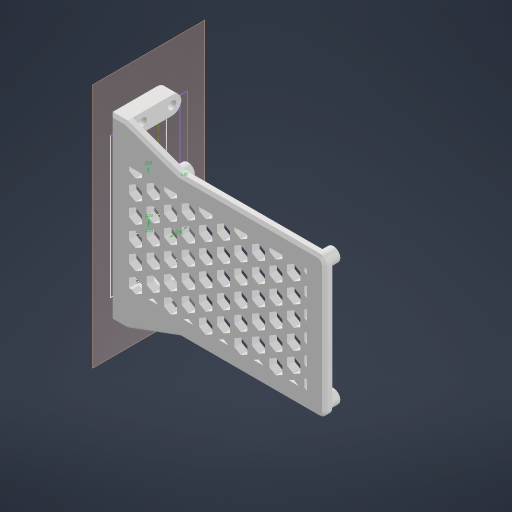
# Autodesk Inventor part: RaspberryPi_baseplate
Saved by Autodesk Inventor 2024 (Build 280153000, 153)
## iProperties
Created: 2025-09-25
Part Number: RaspberryPi_baseplate
Material: Generic
Document SubType Name: Modeling
Designer: kevin
Density: 1 g/cm^3
Appearance: Default
Author: kevin
Autodesk Inventor part; units mm, degrees
(part 1 of 2)
ref_plane "YZ Plane" through (0, 0, 0) normal (1, 0, 0) x (0, 1, 0)
ref_plane "XZ Plane" through (0, 0, 0) normal (0, 1, 0) x (-1, 0, 0)
ref_plane "XY Plane" through (0, 0, 0) normal (0, 0, 1) x (1, 0, 0)
sketch "Sketch1" plane through (0, 0, 0) normal (0, 0, 1) x (1, 0, 0)
  line L0 (-39.5, -28) -> (39.5, -28) projected
  arc A0 (39.5, -28) -> (42.5, -25) centre (39.5, -25) ccw projected
  line L1 (42.5, -25) -> (42.5, 25) projected
  arc A1 (42.5, 25) -> (39.5, 28) centre (39.5, 25) ccw projected
  line L2 (39.5, 28) -> (-39.325, 28) projected
  arc A2 (-39.325, 28) -> (-42.5, 24.825) centre (-39.325, 24.825) ccw projected
  line L3 (-42.5, 24.825) -> (-42.5, -25) projected
  arc A3 (-42.5, -25) -> (-39.5, -28) centre (-39.5, -25) ccw projected
  circle A4 centre (39, 24.5) radius 1.35 construction
  circle A5 centre (39, -24.5) radius 1.35 construction
  circle A6 centre (-19, -24.5) radius 1.35 construction
  circle A7 centre (-19, 24.5) radius 1.35 construction
  circle A8 centre (-19, 24.5) radius 2.75
  circle A9 centre (39, 24.5) radius 2.75
  circle A10 centre (39, -24.5) radius 2.75
  circle A11 centre (-19, -24.5) radius 2.75
  circle A12 centre (-19, -24.5) radius 1.1
  circle A13 centre (-19, 24.5) radius 1.1
  circle A14 centre (39, 24.5) radius 1.1
  circle A15 centre (39, -24.5) radius 1.1
  point P0 (0, 0)
  dimension "d0" = 5.5
  dimension "d1" = 5.5
  dimension "d2" = 5.5
  dimension "d3" = 5.5
  dimension "d4" = 2.2
  dimension "d5" = 2.2
  dimension "d6" = 2.2
  dimension "d7" = 2.2
  constraints: 8 centre point, 8 coincident
  measures "d0" diameter of A8
  measures "d1" diameter of A9
  measures "d2" diameter of A10
  measures "d3" diameter of A11
  measures "d4" diameter of A12
  measures "d5" diameter of A13
  measures "d6" diameter of A14
  measures "d7" diameter of A15
extrude "Extrusion1" add sketch "Sketch1" along normal blind 4 contours A8 | A9 | A10 | A11
sketch "Sketch2" plane through (-19, 24.5, 4) normal (0, 0, 1) x (1, 0, 0)
  circle A0 centre (0, 0) radius 2.75 construction
  circle A1 centre (0, 0) radius 1.1 construction
  circle A2 centre (58, 0) radius 2.75 construction
  circle A3 centre (58, 0) radius 1.1 construction
  circle A4 centre (58, -49) radius 2.75 construction
  circle A5 centre (58, -49) radius 1.1 construction
  circle A6 centre (0, -49) radius 2.75 construction
  circle A7 centre (0, -49) radius 1.1 construction
  line L0 (-20.5, -52.5) -> (58.5, -52.5) projected
  arc A8 (58.5, -52.5) -> (61.5, -49.5) centre (58.5, -49.5) ccw projected
  line L1 (61.5, -49.5) -> (61.5, 0.5) projected
  arc A9 (61.5, 0.5) -> (58.5, 3.5) centre (58.5, 0.5) ccw projected
  line L2 (58.5, 3.5) -> (-20.325, 3.5) projected
  arc A10 (-20.325, 3.5) -> (-23.5, 0.325) centre (-20.325, 0.325) ccw construction
  line L3 (-23.5, 0.325) -> (-23.5, -49.5) projected
  arc A11 (-23.5, -49.5) -> (-20.5, -52.5) centre (-20.5, -49.5) ccw construction
  circle A12 centre (58, 0) radius 1.35 construction
  circle A13 centre (58, -49) radius 1.35 construction
  circle A14 centre (0, -49) radius 1.35 construction
  circle A15 centre (0, 0) radius 1.35 construction
  arc A16 (-3.5, -49) -> (0, -52.5) centre (0, -49) ccw construction
  arc A17 (0, 3.5) -> (-3.5, 0) centre (0, 0) ccw construction
  line L4 (-3.5, 0) -> (-3.5, -49) construction
  line L5 (0, 3.5) -> (58.5, 3.5)
  line L6 (0, -52.5) -> (58.5, -52.5)
  line L7 (54.5, -45.5) -> (3.5, -45.5)
  line L8 (3.5, -45.5) -> (3.5, -3.5) construction
  line L9 (3.5, -3.5) -> (54.5, -3.5)
  line L10 (54.5, -3.5) -> (54.5, -45.5)
  line L11 (3.5, -3.5) -> (54.5, -3.5)
  line L12 (54.5, -45.5) -> (3.5, -45.5)
  line L13 (4.524, -5.8635) -> (7.1369, -4.3549)
  line L14 (7.1369, -4.3549) -> (9.7499, -5.8635)
  line L15 (9.7499, -5.8635) -> (9.7499, -8.8807)
  line L16 (9.7499, -8.8807) -> (7.1369, -10.3893)
  line L17 (7.1369, -10.3893) -> (4.524, -8.8807)
  line L18 (4.524, -8.8807) -> (4.524, -5.8635)
  line L19 (9.7499, -16.8807) -> (7.1369, -18.3893)
  line L20 (9.7499, -13.8635) -> (9.7499, -16.8807)
  line L21 (7.1369, -12.3549) -> (9.7499, -13.8635)
  line L22 (4.524, -13.8635) -> (7.1369, -12.3549)
  line L23 (4.524, -16.8807) -> (4.524, -13.8635)
  line L24 (7.1369, -18.3893) -> (4.524, -16.8807)
  line L25 (9.7499, -24.8807) -> (7.1369, -26.3893)
  line L26 (9.7499, -21.8635) -> (9.7499, -24.8807)
  line L27 (7.1369, -20.3549) -> (9.7499, -21.8635)
  line L28 (4.524, -21.8635) -> (7.1369, -20.3549)
  line L29 (4.524, -24.8807) -> (4.524, -21.8635)
  line L30 (7.1369, -26.3893) -> (4.524, -24.8807)
  line L31 (9.7499, -32.8807) -> (7.1369, -34.3893)
  line L32 (9.7499, -29.8635) -> (9.7499, -32.8807)
  line L33 (7.1369, -28.3549) -> (9.7499, -29.8635)
  line L34 (4.524, -29.8635) -> (7.1369, -28.3549)
  line L35 (4.524, -32.8807) -> (4.524, -29.8635)
  line L36 (7.1369, -34.3893) -> (4.524, -32.8807)
  line L37 (9.7499, -40.8807) -> (7.1369, -42.3893)
  line L38 (9.7499, -37.8635) -> (9.7499, -40.8807)
  line L39 (7.1369, -36.3549) -> (9.7499, -37.8635)
  line L40 (4.524, -37.8635) -> (7.1369, -36.3549)
  line L41 (4.524, -40.8807) -> (4.524, -37.8635)
  line L42 (7.1369, -42.3893) -> (4.524, -40.8807)
  line L43 (16.6781, -12.8807) -> (14.0651, -14.3893)
  line L44 (16.6781, -9.8635) -> (16.6781, -12.8807)
  line L45 (14.0651, -8.3549) -> (16.6781, -9.8635)
  line L46 (11.4522, -9.8635) -> (14.0651, -8.3549)
  line L47 (11.4522, -12.8807) -> (11.4522, -9.8635)
  line L48 (14.0651, -14.3893) -> (11.4522, -12.8807)
  line L49 (16.6781, -20.8807) -> (14.0651, -22.3893)
  line L50 (16.6781, -17.8635) -> (16.6781, -20.8807)
  line L51 (14.0651, -16.3549) -> (16.6781, -17.8635)
  line L52 (11.4522, -17.8635) -> (14.0651, -16.3549)
  line L53 (11.4522, -20.8807) -> (11.4522, -17.8635)
  line L54 (14.0651, -22.3893) -> (11.4522, -20.8807)
  line L55 (16.6781, -28.8807) -> (14.0651, -30.3893)
  line L56 (16.6781, -25.8635) -> (16.6781, -28.8807)
  line L57 (14.0651, -24.3549) -> (16.6781, -25.8635)
  line L58 (11.4522, -25.8635) -> (14.0651, -24.3549)
  line L59 (11.4522, -28.8807) -> (11.4522, -25.8635)
  line L60 (14.0651, -30.3893) -> (11.4522, -28.8807)
  line L61 (16.6781, -36.8807) -> (14.0651, -38.3893)
  line L62 (16.6781, -33.8635) -> (16.6781, -36.8807)
  line L63 (14.0651, -32.3549) -> (16.6781, -33.8635)
  line L64 (11.4522, -33.8635) -> (14.0651, -32.3549)
  line L65 (11.4522, -36.8807) -> (11.4522, -33.8635)
  line L66 (14.0651, -38.3893) -> (11.4522, -36.8807)
  line L67 (16.6781, -44.8807) -> (14.0651, -46.3893)
  line L68 (16.6781, -41.8635) -> (16.6781, -44.8807)
  line L69 (14.0651, -40.3549) -> (16.6781, -41.8635)
  line L70 (11.4522, -41.8635) -> (14.0651, -40.3549)
  line L71 (11.4522, -44.8807) -> (11.4522, -41.8635)
  line L72 (14.0651, -46.3893) -> (11.4522, -44.8807)
  line L73 (16.6781, -4.8807) -> (14.0651, -6.3893)
  line L74 (16.6781, -1.8635) -> (16.6781, -4.8807)
  line L75 (11.4522, -4.8807) -> (11.4522, -1.8635)
  line L76 (14.0651, -0.3549) -> (16.6781, -1.8635) construction
  line L77 (11.4522, -1.8635) -> (14.0651, -0.3549) construction
  line L78 (14.0651, -6.3893) -> (11.4522, -4.8807)
  line L79 (9.7499, -48.8807) -> (7.1369, -50.3893) construction
  line L80 (9.7499, -45.8635) -> (9.7499, -48.8807) construction
  line L81 (7.1369, -44.3549) -> (9.7499, -45.8635)
  line L82 (4.524, -45.8635) -> (7.1369, -44.3549)
  line L83 (4.524, -48.8807) -> (4.524, -45.8635) construction
  line L84 (7.1369, -50.3893) -> (4.524, -48.8807) construction
  line L85 (23.7499, -5.8635) -> (23.7499, -8.8807)
  line L86 (21.1369, -4.3549) -> (23.7499, -5.8635)
  line L87 (18.524, -5.8635) -> (21.1369, -4.3549)
  line L88 (18.524, -8.8807) -> (18.524, -5.8635)
  line L89 (21.1369, -10.3893) -> (18.524, -8.8807)
  line L90 (23.7499, -8.8807) -> (21.1369, -10.3893)
  line L91 (18.524, -40.8807) -> (18.524, -37.8635)
  line L92 (21.1369, -42.3893) -> (18.524, -40.8807)
  line L93 (23.7499, -37.8635) -> (23.7499, -40.8807)
  line L94 (23.7499, -40.8807) -> (21.1369, -42.3893)
  line L95 (25.4522, -20.8807) -> (25.4522, -17.8635)
  line L96 (25.4522, -17.8635) -> (28.0651, -16.3549)
  line L97 (28.0651, -14.3893) -> (25.4522, -12.8807)
  line L98 (30.6781, -12.8807) -> (28.0651, -14.3893)
  line L99 (28.0651, -16.3549) -> (30.6781, -17.8635)
  line L100 (28.0651, -22.3893) -> (25.4522, -20.8807)
  line L101 (30.6781, -17.8635) -> (30.6781, -20.8807)
  line L102 (30.6781, -20.8807) -> (28.0651, -22.3893)
  line L103 (25.4522, -41.8635) -> (28.0651, -40.3549)
  line L104 (28.0651, -40.3549) -> (30.6781, -41.8635)
  line L105 (25.4522, -25.8635) -> (28.0651, -24.3549)
  line L106 (28.0651, -24.3549) -> (30.6781, -25.8635)
  line L107 (30.6781, -25.8635) -> (30.6781, -28.8807)
  line L108 (30.6781, -28.8807) -> (28.0651, -30.3893)
  line L109 (28.0651, -30.3893) -> (25.4522, -28.8807)
  line L110 (28.0651, -32.3549) -> (30.6781, -33.8635)
  line L111 (25.4522, -33.8635) -> (28.0651, -32.3549)
  line L112 (30.6781, -33.8635) -> (30.6781, -36.8807)
  line L113 (25.4522, -36.8807) -> (25.4522, -33.8635)
  line L114 (30.6781, -36.8807) -> (28.0651, -38.3893)
  line L115 (28.0651, -38.3893) -> (25.4522, -36.8807)
  line L116 (25.4522, -28.8807) -> (25.4522, -25.8635)
  line L117 (23.7499, -24.8807) -> (21.1369, -26.3893)
  line L118 (23.7499, -21.8635) -> (23.7499, -24.8807)
  line L119 (21.1369, -20.3549) -> (23.7499, -21.8635)
  line L120 (18.524, -21.8635) -> (21.1369, -20.3549)
  line L121 (18.524, -24.8807) -> (18.524, -21.8635)
  line L122 (21.1369, -26.3893) -> (18.524, -24.8807)
  line L123 (23.7499, -32.8807) -> (21.1369, -34.3893)
  line L124 (18.524, -37.8635) -> (21.1369, -36.3549)
  line L125 (21.1369, -36.3549) -> (23.7499, -37.8635)
  line L126 (21.1369, -34.3893) -> (18.524, -32.8807)
  line L127 (23.7499, -29.8635) -> (23.7499, -32.8807)
  line L128 (18.524, -32.8807) -> (18.524, -29.8635)
  line L129 (21.1369, -28.3549) -> (23.7499, -29.8635)
  line L130 (18.524, -29.8635) -> (21.1369, -28.3549)
  line L131 (23.7499, -16.8807) -> (21.1369, -18.3893)
  line L132 (23.7499, -13.8635) -> (23.7499, -16.8807)
  line L133 (21.1369, -18.3893) -> (18.524, -16.8807)
  line L134 (21.1369, -12.3549) -> (23.7499, -13.8635)
  line L135 (18.524, -16.8807) -> (18.524, -13.8635)
  line L136 (18.524, -13.8635) -> (21.1369, -12.3549)
  line L137 (30.6781, -9.8635) -> (30.6781, -12.8807)
  line L138 (28.0651, -8.3549) -> (30.6781, -9.8635)
  line L139 (25.4522, -9.8635) -> (28.0651, -8.3549)
  line L140 (25.4522, -12.8807) -> (25.4522, -9.8635)
  line L141 (28.0651, -6.3893) -> (25.4522, -4.8807)
  line L142 (30.6781, -4.8807) -> (28.0651, -6.3893)
  line L143 (30.6781, -1.8635) -> (30.6781, -4.8807)
  line L144 (28.0651, -0.3549) -> (30.6781, -1.8635) construction
  line L145 (25.4522, -1.8635) -> (28.0651, -0.3549) construction
  line L146 (25.4522, -4.8807) -> (25.4522, -1.8635)
  line L147 (25.4522, -44.8807) -> (25.4522, -41.8635)
  line L148 (28.0651, -46.3893) -> (25.4522, -44.8807)
  line L149 (30.6781, -44.8807) -> (28.0651, -46.3893)
  line L150 (30.6781, -41.8635) -> (30.6781, -44.8807)
  line L151 (21.1369, -44.3549) -> (23.7499, -45.8635)
  line L152 (18.524, -45.8635) -> (21.1369, -44.3549)
  line L153 (18.524, -48.8807) -> (18.524, -45.8635) construction
  line L154 (21.1369, -50.3893) -> (18.524, -48.8807) construction
  line L155 (23.7499, -48.8807) -> (21.1369, -50.3893) construction
  line L156 (23.7499, -45.8635) -> (23.7499, -48.8807) construction
  line L157 (37.7499, -5.8635) -> (37.7499, -8.8807)
  line L158 (35.1369, -4.3549) -> (37.7499, -5.8635)
  line L159 (32.524, -5.8635) -> (35.1369, -4.3549)
  line L160 (32.524, -8.8807) -> (32.524, -5.8635)
  line L161 (35.1369, -10.3893) -> (32.524, -8.8807)
  line L162 (37.7499, -8.8807) -> (35.1369, -10.3893)
  line L163 (32.524, -40.8807) -> (32.524, -37.8635)
  line L164 (35.1369, -42.3893) -> (32.524, -40.8807)
  line L165 (37.7499, -37.8635) -> (37.7499, -40.8807)
  line L166 (37.7499, -40.8807) -> (35.1369, -42.3893)
  line L167 (39.4522, -20.8807) -> (39.4522, -17.8635)
  line L168 (39.4522, -17.8635) -> (42.0651, -16.3549)
  line L169 (42.0651, -14.3893) -> (39.4522, -12.8807)
  line L170 (44.6781, -12.8807) -> (42.0651, -14.3893)
  line L171 (42.0651, -16.3549) -> (44.6781, -17.8635)
  line L172 (42.0651, -22.3893) -> (39.4522, -20.8807)
  line L173 (44.6781, -17.8635) -> (44.6781, -20.8807)
  line L174 (44.6781, -20.8807) -> (42.0651, -22.3893)
  line L175 (39.4522, -41.8635) -> (42.0651, -40.3549)
  line L176 (42.0651, -40.3549) -> (44.6781, -41.8635)
  line L177 (39.4522, -25.8635) -> (42.0651, -24.3549)
  line L178 (42.0651, -24.3549) -> (44.6781, -25.8635)
  line L179 (44.6781, -25.8635) -> (44.6781, -28.8807)
  line L180 (44.6781, -28.8807) -> (42.0651, -30.3893)
  line L181 (42.0651, -30.3893) -> (39.4522, -28.8807)
  line L182 (42.0651, -32.3549) -> (44.6781, -33.8635)
  line L183 (39.4522, -33.8635) -> (42.0651, -32.3549)
  line L184 (44.6781, -33.8635) -> (44.6781, -36.8807)
  line L185 (39.4522, -36.8807) -> (39.4522, -33.8635)
  line L186 (44.6781, -36.8807) -> (42.0651, -38.3893)
  line L187 (42.0651, -38.3893) -> (39.4522, -36.8807)
  line L188 (39.4522, -28.8807) -> (39.4522, -25.8635)
  line L189 (37.7499, -24.8807) -> (35.1369, -26.3893)
  line L190 (37.7499, -21.8635) -> (37.7499, -24.8807)
  line L191 (35.1369, -20.3549) -> (37.7499, -21.8635)
  line L192 (32.524, -21.8635) -> (35.1369, -20.3549)
  line L193 (32.524, -24.8807) -> (32.524, -21.8635)
  line L194 (35.1369, -26.3893) -> (32.524, -24.8807)
  line L195 (37.7499, -32.8807) -> (35.1369, -34.3893)
  line L196 (32.524, -37.8635) -> (35.1369, -36.3549)
  line L197 (35.1369, -36.3549) -> (37.7499, -37.8635)
  line L198 (35.1369, -34.3893) -> (32.524, -32.8807)
  line L199 (37.7499, -29.8635) -> (37.7499, -32.8807)
  line L200 (32.524, -32.8807) -> (32.524, -29.8635)
  line L201 (35.1369, -28.3549) -> (37.7499, -29.8635)
  line L202 (32.524, -29.8635) -> (35.1369, -28.3549)
  line L203 (37.7499, -16.8807) -> (35.1369, -18.3893)
  line L204 (37.7499, -13.8635) -> (37.7499, -16.8807)
  line L205 (35.1369, -18.3893) -> (32.524, -16.8807)
  line L206 (35.1369, -12.3549) -> (37.7499, -13.8635)
  line L207 (32.524, -16.8807) -> (32.524, -13.8635)
  line L208 (32.524, -13.8635) -> (35.1369, -12.3549)
  line L209 (44.6781, -9.8635) -> (44.6781, -12.8807)
  line L210 (42.0651, -8.3549) -> (44.6781, -9.8635)
  line L211 (39.4522, -9.8635) -> (42.0651, -8.3549)
  line L212 (39.4522, -12.8807) -> (39.4522, -9.8635)
  line L213 (42.0651, -6.3893) -> (39.4522, -4.8807)
  line L214 (44.6781, -4.8807) -> (42.0651, -6.3893)
  line L215 (44.6781, -1.8635) -> (44.6781, -4.8807)
  line L216 (42.0651, -0.3549) -> (44.6781, -1.8635) construction
  line L217 (39.4522, -1.8635) -> (42.0651, -0.3549) construction
  line L218 (39.4522, -4.8807) -> (39.4522, -1.8635)
  line L219 (39.4522, -44.8807) -> (39.4522, -41.8635)
  line L220 (42.0651, -46.3893) -> (39.4522, -44.8807)
  line L221 (44.6781, -44.8807) -> (42.0651, -46.3893)
  line L222 (44.6781, -41.8635) -> (44.6781, -44.8807)
  line L223 (35.1369, -44.3549) -> (37.7499, -45.8635)
  line L224 (32.524, -45.8635) -> (35.1369, -44.3549)
  line L225 (32.524, -48.8807) -> (32.524, -45.8635) construction
  line L226 (35.1369, -50.3893) -> (32.524, -48.8807) construction
  line L227 (37.7499, -48.8807) -> (35.1369, -50.3893) construction
  line L228 (37.7499, -45.8635) -> (37.7499, -48.8807) construction
  line L229 (51.7499, -5.8635) -> (51.7499, -8.8807)
  line L230 (49.1369, -4.3549) -> (51.7499, -5.8635)
  line L231 (46.524, -5.8635) -> (49.1369, -4.3549)
  line L232 (46.524, -8.8807) -> (46.524, -5.8635)
  line L233 (49.1369, -10.3893) -> (46.524, -8.8807)
  line L234 (51.7499, -8.8807) -> (49.1369, -10.3893)
  line L235 (46.524, -40.8807) -> (46.524, -37.8635)
  line L236 (49.1369, -42.3893) -> (46.524, -40.8807)
  line L237 (51.7499, -37.8635) -> (51.7499, -40.8807)
  line L238 (51.7499, -40.8807) -> (49.1369, -42.3893)
  line L239 (53.4522, -20.8807) -> (53.4522, -17.8635)
  line L240 (53.4522, -17.8635) -> (56.0651, -16.3549)
  line L241 (56.0651, -14.3893) -> (53.4522, -12.8807)
  line L242 (58.6781, -12.8807) -> (56.0651, -14.3893) construction
  line L243 (56.0651, -16.3549) -> (58.6781, -17.8635) construction
  line L244 (56.0651, -22.3893) -> (53.4522, -20.8807)
  line L245 (58.6781, -17.8635) -> (58.6781, -20.8807) construction
  line L246 (58.6781, -20.8807) -> (56.0651, -22.3893) construction
  line L247 (53.4522, -41.8635) -> (56.0651, -40.3549)
  line L248 (56.0651, -40.3549) -> (58.6781, -41.8635) construction
  line L249 (53.4522, -25.8635) -> (56.0651, -24.3549)
  line L250 (56.0651, -24.3549) -> (58.6781, -25.8635) construction
  line L251 (58.6781, -25.8635) -> (58.6781, -28.8807) construction
  line L252 (58.6781, -28.8807) -> (56.0651, -30.3893) construction
  line L253 (56.0651, -30.3893) -> (53.4522, -28.8807)
  line L254 (56.0651, -32.3549) -> (58.6781, -33.8635) construction
  line L255 (53.4522, -33.8635) -> (56.0651, -32.3549)
  line L256 (58.6781, -33.8635) -> (58.6781, -36.8807) construction
  line L257 (53.4522, -36.8807) -> (53.4522, -33.8635)
  line L258 (58.6781, -36.8807) -> (56.0651, -38.3893) construction
  line L259 (56.0651, -38.3893) -> (53.4522, -36.8807)
  line L260 (53.4522, -28.8807) -> (53.4522, -25.8635)
  line L261 (51.7499, -24.8807) -> (49.1369, -26.3893)
  line L262 (51.7499, -21.8635) -> (51.7499, -24.8807)
  line L263 (49.1369, -20.3549) -> (51.7499, -21.8635)
  line L264 (46.524, -21.8635) -> (49.1369, -20.3549)
  line L265 (46.524, -24.8807) -> (46.524, -21.8635)
  line L266 (49.1369, -26.3893) -> (46.524, -24.8807)
  line L267 (51.7499, -32.8807) -> (49.1369, -34.3893)
  line L268 (46.524, -37.8635) -> (49.1369, -36.3549)
  line L269 (49.1369, -36.3549) -> (51.7499, -37.8635)
  line L270 (49.1369, -34.3893) -> (46.524, -32.8807)
  line L271 (51.7499, -29.8635) -> (51.7499, -32.8807)
  line L272 (46.524, -32.8807) -> (46.524, -29.8635)
  line L273 (49.1369, -28.3549) -> (51.7499, -29.8635)
  line L274 (46.524, -29.8635) -> (49.1369, -28.3549)
  line L275 (51.7499, -16.8807) -> (49.1369, -18.3893)
  line L276 (51.7499, -13.8635) -> (51.7499, -16.8807)
  line L277 (49.1369, -18.3893) -> (46.524, -16.8807)
  line L278 (49.1369, -12.3549) -> (51.7499, -13.8635)
  line L279 (46.524, -16.8807) -> (46.524, -13.8635)
  line L280 (46.524, -13.8635) -> (49.1369, -12.3549)
  line L281 (58.6781, -9.8635) -> (58.6781, -12.8807) construction
  line L282 (56.0651, -8.3549) -> (58.6781, -9.8635) construction
  line L283 (53.4522, -9.8635) -> (56.0651, -8.3549)
  line L284 (53.4522, -12.8807) -> (53.4522, -9.8635)
  line L285 (56.0651, -6.3893) -> (53.4522, -4.8807)
  line L286 (58.6781, -4.8807) -> (56.0651, -6.3893) construction
  line L287 (58.6781, -1.8635) -> (58.6781, -4.8807) construction
  line L288 (56.0651, -0.3549) -> (58.6781, -1.8635)
  line L289 (53.4522, -1.8635) -> (56.0651, -0.3549)
  line L290 (53.4522, -4.8807) -> (53.4522, -1.8635)
  line L291 (53.4522, -44.8807) -> (53.4522, -41.8635)
  line L292 (56.0651, -46.3893) -> (53.4522, -44.8807)
  line L293 (58.6781, -44.8807) -> (56.0651, -46.3893)
  line L294 (58.6781, -41.8635) -> (58.6781, -44.8807) construction
  line L295 (49.1369, -44.3549) -> (51.7499, -45.8635)
  line L296 (46.524, -45.8635) -> (49.1369, -44.3549)
  line L297 (46.524, -48.8807) -> (46.524, -45.8635) construction
  line L298 (49.1369, -50.3893) -> (46.524, -48.8807) construction
  line L299 (51.7499, -48.8807) -> (49.1369, -50.3893) construction
  line L300 (51.7499, -45.8635) -> (51.7499, -48.8807) construction
  line L301 (65.7499, -5.8635) -> (65.7499, -8.8807) construction
  line L302 (63.1369, -4.3549) -> (65.7499, -5.8635) construction
  line L303 (60.524, -5.8635) -> (63.1369, -4.3549) construction
  line L304 (60.524, -8.8807) -> (60.524, -5.8635)
  line L305 (63.1369, -10.3893) -> (60.524, -8.8807) construction
  line L306 (65.7499, -8.8807) -> (63.1369, -10.3893) construction
  line L307 (60.524, -40.8807) -> (60.524, -37.8635)
  line L308 (63.1369, -42.3893) -> (60.524, -40.8807) construction
  line L309 (65.7499, -37.8635) -> (65.7499, -40.8807) construction
  line L310 (65.7499, -40.8807) -> (63.1369, -42.3893) construction
  line L311 (67.4522, -20.8807) -> (67.4522, -17.8635) construction
  line L312 (67.4522, -17.8635) -> (70.0651, -16.3549) construction
  line L313 (70.0651, -14.3893) -> (67.4522, -12.8807) construction
  line L314 (72.6781, -12.8807) -> (70.0651, -14.3893) construction
  line L315 (70.0651, -16.3549) -> (72.6781, -17.8635) construction
  line L316 (70.0651, -22.3893) -> (67.4522, -20.8807) construction
  line L317 (72.6781, -17.8635) -> (72.6781, -20.8807) construction
  line L318 (72.6781, -20.8807) -> (70.0651, -22.3893) construction
  line L319 (67.4522, -41.8635) -> (70.0651, -40.3549) construction
  line L320 (70.0651, -40.3549) -> (72.6781, -41.8635) construction
  line L321 (67.4522, -25.8635) -> (70.0651, -24.3549) construction
  line L322 (70.0651, -24.3549) -> (72.6781, -25.8635) construction
  line L323 (72.6781, -25.8635) -> (72.6781, -28.8807) construction
  line L324 (72.6781, -28.8807) -> (70.0651, -30.3893) construction
  line L325 (70.0651, -30.3893) -> (67.4522, -28.8807) construction
  line L326 (70.0651, -32.3549) -> (72.6781, -33.8635) construction
  line L327 (67.4522, -33.8635) -> (70.0651, -32.3549) construction
  line L328 (72.6781, -33.8635) -> (72.6781, -36.8807) construction
  line L329 (67.4522, -36.8807) -> (67.4522, -33.8635) construction
  line L330 (72.6781, -36.8807) -> (70.0651, -38.3893) construction
  line L331 (70.0651, -38.3893) -> (67.4522, -36.8807) construction
  line L332 (67.4522, -28.8807) -> (67.4522, -25.8635) construction
  line L333 (65.7499, -24.8807) -> (63.1369, -26.3893) construction
  line L334 (65.7499, -21.8635) -> (65.7499, -24.8807) construction
  line L335 (63.1369, -20.3549) -> (65.7499, -21.8635) construction
  line L336 (60.524, -21.8635) -> (63.1369, -20.3549) construction
  line L337 (60.524, -24.8807) -> (60.524, -21.8635)
  line L338 (63.1369, -26.3893) -> (60.524, -24.8807) construction
  line L339 (65.7499, -32.8807) -> (63.1369, -34.3893) construction
  line L340 (60.524, -37.8635) -> (63.1369, -36.3549) construction
  line L341 (63.1369, -36.3549) -> (65.7499, -37.8635) construction
  line L342 (63.1369, -34.3893) -> (60.524, -32.8807) construction
  line L343 (65.7499, -29.8635) -> (65.7499, -32.8807) construction
  line L344 (60.524, -32.8807) -> (60.524, -29.8635)
  line L345 (63.1369, -28.3549) -> (65.7499, -29.8635) construction
  line L346 (60.524, -29.8635) -> (63.1369, -28.3549) construction
  line L347 (65.7499, -16.8807) -> (63.1369, -18.3893) construction
  line L348 (65.7499, -13.8635) -> (65.7499, -16.8807) construction
  line L349 (63.1369, -18.3893) -> (60.524, -16.8807) construction
  line L350 (63.1369, -12.3549) -> (65.7499, -13.8635) construction
  line L351 (60.524, -16.8807) -> (60.524, -13.8635)
  line L352 (60.524, -13.8635) -> (63.1369, -12.3549) construction
  line L353 (72.6781, -9.8635) -> (72.6781, -12.8807) construction
  line L354 (70.0651, -8.3549) -> (72.6781, -9.8635) construction
  line L355 (67.4522, -9.8635) -> (70.0651, -8.3549) construction
  line L356 (67.4522, -12.8807) -> (67.4522, -9.8635) construction
  line L357 (70.0651, -6.3893) -> (67.4522, -4.8807) construction
  line L358 (72.6781, -4.8807) -> (70.0651, -6.3893) construction
  line L359 (72.6781, -1.8635) -> (72.6781, -4.8807) construction
  line L360 (70.0651, -0.3549) -> (72.6781, -1.8635) construction
  line L361 (67.4522, -1.8635) -> (70.0651, -0.3549) construction
  line L362 (67.4522, -4.8807) -> (67.4522, -1.8635) construction
  line L363 (67.4522, -44.8807) -> (67.4522, -41.8635) construction
  line L364 (70.0651, -46.3893) -> (67.4522, -44.8807) construction
  line L365 (72.6781, -44.8807) -> (70.0651, -46.3893) construction
  line L366 (72.6781, -41.8635) -> (72.6781, -44.8807) construction
  line L367 (63.1369, -44.3549) -> (65.7499, -45.8635) construction
  line L368 (60.524, -45.8635) -> (63.1369, -44.3549) construction
  line L369 (60.524, -48.8807) -> (60.524, -45.8635)
  line L370 (63.1369, -50.3893) -> (60.524, -48.8807) construction
  line L371 (65.7499, -48.8807) -> (63.1369, -50.3893) construction
  line L372 (65.7499, -45.8635) -> (65.7499, -48.8807) construction
  line L373 (79.7499, -5.8635) -> (79.7499, -8.8807) construction
  line L374 (77.1369, -4.3549) -> (79.7499, -5.8635) construction
  line L375 (74.524, -5.8635) -> (77.1369, -4.3549) construction
  line L376 (74.524, -8.8807) -> (74.524, -5.8635) construction
  line L377 (77.1369, -10.3893) -> (74.524, -8.8807) construction
  line L378 (79.7499, -8.8807) -> (77.1369, -10.3893) construction
  line L379 (74.524, -40.8807) -> (74.524, -37.8635) construction
  line L380 (77.1369, -42.3893) -> (74.524, -40.8807) construction
  line L381 (79.7499, -37.8635) -> (79.7499, -40.8807) construction
  line L382 (79.7499, -40.8807) -> (77.1369, -42.3893) construction
  line L383 (81.4522, -20.8807) -> (81.4522, -17.8635) construction
  line L384 (81.4522, -17.8635) -> (84.0651, -16.3549) construction
  line L385 (84.0651, -14.3893) -> (81.4522, -12.8807) construction
  line L386 (86.6781, -12.8807) -> (84.0651, -14.3893) construction
  line L387 (84.0651, -16.3549) -> (86.6781, -17.8635) construction
  line L388 (84.0651, -22.3893) -> (81.4522, -20.8807) construction
  line L389 (86.6781, -17.8635) -> (86.6781, -20.8807) construction
  line L390 (86.6781, -20.8807) -> (84.0651, -22.3893) construction
  line L391 (81.4522, -41.8635) -> (84.0651, -40.3549) construction
  line L392 (84.0651, -40.3549) -> (86.6781, -41.8635) construction
  line L393 (81.4522, -25.8635) -> (84.0651, -24.3549) construction
  line L394 (84.0651, -24.3549) -> (86.6781, -25.8635) construction
  line L395 (86.6781, -25.8635) -> (86.6781, -28.8807) construction
  line L396 (86.6781, -28.8807) -> (84.0651, -30.3893) construction
  line L397 (84.0651, -30.3893) -> (81.4522, -28.8807) construction
  line L398 (84.0651, -32.3549) -> (86.6781, -33.8635) construction
  line L399 (81.4522, -33.8635) -> (84.0651, -32.3549) construction
  line L400 (86.6781, -33.8635) -> (86.6781, -36.8807) construction
  line L401 (81.4522, -36.8807) -> (81.4522, -33.8635) construction
  line L402 (86.6781, -36.8807) -> (84.0651, -38.3893) construction
  line L403 (84.0651, -38.3893) -> (81.4522, -36.8807) construction
  line L404 (81.4522, -28.8807) -> (81.4522, -25.8635) construction
  line L405 (79.7499, -24.8807) -> (77.1369, -26.3893) construction
  line L406 (79.7499, -21.8635) -> (79.7499, -24.8807) construction
  line L407 (77.1369, -20.3549) -> (79.7499, -21.8635) construction
  line L408 (74.524, -21.8635) -> (77.1369, -20.3549) construction
  line L409 (74.524, -24.8807) -> (74.524, -21.8635) construction
  line L410 (77.1369, -26.3893) -> (74.524, -24.8807) construction
  line L411 (79.7499, -32.8807) -> (77.1369, -34.3893) construction
  line L412 (74.524, -37.8635) -> (77.1369, -36.3549) construction
  line L413 (77.1369, -36.3549) -> (79.7499, -37.8635) construction
  line L414 (77.1369, -34.3893) -> (74.524, -32.8807) construction
  line L415 (79.7499, -29.8635) -> (79.7499, -32.8807) construction
  line L416 (74.524, -32.8807) -> (74.524, -29.8635) construction
  line L417 (77.1369, -28.3549) -> (79.7499, -29.8635) construction
  line L418 (74.524, -29.8635) -> (77.1369, -28.3549) construction
  line L419 (79.7499, -16.8807) -> (77.1369, -18.3893) construction
  line L420 (79.7499, -13.8635) -> (79.7499, -16.8807) construction
  line L421 (77.1369, -18.3893) -> (74.524, -16.8807) construction
  line L422 (77.1369, -12.3549) -> (79.7499, -13.8635) construction
  line L423 (74.524, -16.8807) -> (74.524, -13.8635) construction
  line L424 (74.524, -13.8635) -> (77.1369, -12.3549) construction
  line L425 (86.6781, -9.8635) -> (86.6781, -12.8807) construction
  line L426 (84.0651, -8.3549) -> (86.6781, -9.8635) construction
  line L427 (81.4522, -9.8635) -> (84.0651, -8.3549) construction
  line L428 (81.4522, -12.8807) -> (81.4522, -9.8635) construction
  line L429 (84.0651, -6.3893) -> (81.4522, -4.8807) construction
  line L430 (86.6781, -4.8807) -> (84.0651, -6.3893) construction
  line L431 (86.6781, -1.8635) -> (86.6781, -4.8807) construction
  line L432 (84.0651, -0.3549) -> (86.6781, -1.8635) construction
  line L433 (81.4522, -1.8635) -> (84.0651, -0.3549) construction
  line L434 (81.4522, -4.8807) -> (81.4522, -1.8635) construction
  line L435 (81.4522, -44.8807) -> (81.4522, -41.8635) construction
  line L436 (84.0651, -46.3893) -> (81.4522, -44.8807) construction
  line L437 (86.6781, -44.8807) -> (84.0651, -46.3893) construction
  line L438 (86.6781, -41.8635) -> (86.6781, -44.8807) construction
  line L439 (77.1369, -44.3549) -> (79.7499, -45.8635) construction
  line L440 (74.524, -45.8635) -> (77.1369, -44.3549) construction
  line L441 (74.524, -48.8807) -> (74.524, -45.8635) construction
  line L442 (77.1369, -50.3893) -> (74.524, -48.8807) construction
  line L443 (79.7499, -48.8807) -> (77.1369, -50.3893) construction
  line L444 (79.7499, -45.8635) -> (79.7499, -48.8807) construction
  line L445 (-13.5, 3.5) -> (-13.5, -52.5) construction
  line L446 (-13.5, 3.5) -> (0, 3.5)
  line L447 (-23.5, -52.5) -> (0, -52.5)
  line L448 (-16.5, -45.5) -> (-16.5, -3.5)
  line L449 (-16.5, -3.5) -> (54.5, -3.5)
  line L450 (54.5, -3.5) -> (54.5, -45.5)
  line L451 (54.5, -45.5) -> (-16.5, -45.5)
  line L452 (-23.5, -15.3721) -> (-23.5, 3.5)
  line L453 (-16.7764, 3.5) -> (-23.5, 3.5)
  line L454 (-23.5, -49.5) -> (-23.5, -52.5)
  line L455 (2.6781, -9.8635) -> (2.6781, -12.8807)
  line L456 (2.6781, -12.8807) -> (0.0651, -14.3893)
  line L457 (0.0651, -8.3549) -> (2.6781, -9.8635)
  line L458 (0.0651, -16.3549) -> (2.6781, -17.8635)
  line L459 (2.6781, -17.8635) -> (2.6781, -20.8807)
  line L460 (2.6781, -20.8807) -> (0.0651, -22.3893)
  line L461 (-2.5478, -9.8635) -> (0.0651, -8.3549)
  line L462 (-2.5478, -12.8807) -> (-2.5478, -9.8635)
  line L463 (0.0651, -14.3893) -> (-2.5478, -12.8807)
  line L464 (0.0651, -22.3893) -> (-2.5478, -20.8807)
  line L465 (-2.5478, -20.8807) -> (-2.5478, -17.8635)
  line L466 (-2.5478, -17.8635) -> (0.0651, -16.3549)
  line L467 (-4.2501, -24.8807) -> (-6.8631, -26.3893)
  line L468 (-4.2501, -13.8635) -> (-4.2501, -16.8807)
  line L469 (-6.8631, -12.3549) -> (-4.2501, -13.8635)
  line L470 (-4.2501, -16.8807) -> (-6.8631, -18.3893)
  line L471 (-9.476, -8.8807) -> (-9.476, -5.8635)
  line L472 (-6.8631, -10.3893) -> (-9.476, -8.8807)
  line L473 (-6.8631, -18.3893) -> (-9.476, -16.8807)
  line L474 (-9.476, -16.8807) -> (-9.476, -13.8635)
  line L475 (-9.476, -13.8635) -> (-6.8631, -12.3549)
  line L476 (-4.2501, -5.8635) -> (-4.2501, -8.8807)
  line L477 (-6.8631, -4.3549) -> (-4.2501, -5.8635)
  line L478 (-4.2501, -8.8807) -> (-6.8631, -10.3893)
  line L479 (-9.476, -5.8635) -> (-6.8631, -4.3549)
  line L480 (2.6781, -25.8635) -> (2.6781, -28.8807)
  line L481 (0.0651, -24.3549) -> (2.6781, -25.8635)
  line L482 (2.6781, -28.8807) -> (0.0651, -30.3893)
  line L483 (-2.5478, -25.8635) -> (0.0651, -24.3549)
  line L484 (2.6781, -33.8635) -> (2.6781, -36.8807)
  line L485 (0.0651, -32.3549) -> (2.6781, -33.8635)
  line L486 (-2.5478, -28.8807) -> (-2.5478, -25.8635)
  line L487 (0.0651, -30.3893) -> (-2.5478, -28.8807)
  line L488 (-2.5478, -33.8635) -> (0.0651, -32.3549)
  line L489 (-2.5478, -36.8807) -> (-2.5478, -33.8635)
  line L490 (-6.8631, -26.3893) -> (-9.476, -24.8807)
  line L491 (-4.2501, -21.8635) -> (-4.2501, -24.8807)
  line L492 (-4.2501, -29.8635) -> (-4.2501, -32.8807)
  line L493 (-4.2501, -32.8807) -> (-6.8631, -34.3893)
  line L494 (-6.8631, -20.3549) -> (-4.2501, -21.8635)
  line L495 (-6.8631, -28.3549) -> (-4.2501, -29.8635)
  line L496 (-9.476, -29.8635) -> (-6.8631, -28.3549)
  line L497 (-9.476, -24.8807) -> (-9.476, -21.8635)
  line L498 (-9.476, -21.8635) -> (-6.8631, -20.3549)
  line L499 (-4.2501, -37.8635) -> (-4.2501, -40.8807)
  line L500 (-6.8631, -36.3549) -> (-4.2501, -37.8635)
  line L501 (-4.2501, -40.8807) -> (-6.8631, -42.3893)
  line L502 (-9.476, -32.8807) -> (-9.476, -29.8635)
  line L503 (-6.8631, -34.3893) -> (-9.476, -32.8807)
  line L504 (-9.476, -37.8635) -> (-6.8631, -36.3549)
  line L505 (-9.476, -40.8807) -> (-9.476, -37.8635)
  line L506 (-6.8631, -42.3893) -> (-9.476, -40.8807)
  line L507 (2.6781, -36.8807) -> (0.0651, -38.3893)
  line L508 (0.0651, -38.3893) -> (-2.5478, -36.8807)
  line L509 (2.6781, -44.8807) -> (0.0651, -46.3893)
  line L510 (2.6781, -41.8635) -> (2.6781, -44.8807)
  line L511 (0.0651, -40.3549) -> (2.6781, -41.8635)
  line L512 (-2.5478, -41.8635) -> (0.0651, -40.3549)
  line L513 (-2.5478, -44.8807) -> (-2.5478, -41.8635)
  line L514 (0.0651, -46.3893) -> (-2.5478, -44.8807)
  line L515 (-6.8631, -44.3549) -> (-4.2501, -45.8635)
  line L516 (2.6781, -4.8807) -> (0.0651, -6.3893)
  line L517 (0.0651, -6.3893) -> (-2.5478, -4.8807)
  line L518 (2.6781, -1.8635) -> (2.6781, -4.8807)
  line L519 (-2.5478, -4.8807) -> (-2.5478, -1.8635)
  line L520 (0.0651, -0.3549) -> (2.6781, -1.8635) construction
  line L521 (-2.5478, -1.8635) -> (0.0651, -0.3549) construction
  line L522 (4.524, -16.8807) -> (4.524, -13.8635)
  line L523 (4.524, -8.8807) -> (4.524, -5.8635)
  line L524 (-9.476, -45.8635) -> (-6.8631, -44.3549)
  line L525 (-9.476, -48.8807) -> (-9.476, -45.8635) construction
  line L526 (-4.2501, -45.8635) -> (-4.2501, -48.8807) construction
  line L527 (-4.2501, -48.8807) -> (-6.8631, -50.3893) construction
  line L528 (-6.8631, -50.3893) -> (-9.476, -48.8807) construction
  line L529 (-11.3219, -9.8635) -> (-11.3219, -12.8807)
  line L530 (-11.3219, -12.8807) -> (-13.9349, -14.3893)
  line L531 (-13.9349, -8.3549) -> (-11.3219, -9.8635)
  line L532 (-13.9349, -16.3549) -> (-11.3219, -17.8635)
  line L533 (-11.3219, -17.8635) -> (-11.3219, -20.8807)
  line L534 (-11.3219, -20.8807) -> (-13.9349, -22.3893)
  line L535 (-16.5478, -9.8635) -> (-13.9349, -8.3549)
  line L536 (-16.5478, -12.8807) -> (-16.5478, -9.8635)
  line L537 (-13.9349, -14.3893) -> (-16.5478, -12.8807)
  line L538 (-13.9349, -22.3893) -> (-16.5478, -20.8807)
  line L539 (-16.5478, -20.8807) -> (-16.5478, -17.8635)
  line L540 (-16.5478, -17.8635) -> (-13.9349, -16.3549)
  line L541 (-18.2501, -24.8807) -> (-20.8631, -26.3893) construction
  line L542 (-18.2501, -13.8635) -> (-18.2501, -16.8807) construction
  line L543 (-20.8631, -12.3549) -> (-18.2501, -13.8635) construction
  line L544 (-18.2501, -16.8807) -> (-20.8631, -18.3893) construction
  line L545 (-23.476, -8.8807) -> (-23.476, -5.8635)
  line L546 (-20.8631, -10.3893) -> (-23.476, -8.8807) construction
  line L547 (-20.8631, -18.3893) -> (-23.476, -16.8807) construction
  line L548 (-23.476, -16.8807) -> (-23.476, -13.8635)
  line L549 (-23.476, -13.8635) -> (-20.8631, -12.3549) construction
  line L550 (-18.2501, -5.8635) -> (-18.2501, -8.8807) construction
  line L551 (-20.8631, -4.3549) -> (-18.2501, -5.8635) construction
  line L552 (-18.2501, -8.8807) -> (-20.8631, -10.3893) construction
  line L553 (-23.476, -5.8635) -> (-20.8631, -4.3549) construction
  line L554 (-11.3219, -25.8635) -> (-11.3219, -28.8807)
  line L555 (-13.9349, -24.3549) -> (-11.3219, -25.8635)
  line L556 (-11.3219, -28.8807) -> (-13.9349, -30.3893)
  line L557 (-16.5478, -25.8635) -> (-13.9349, -24.3549)
  line L558 (-11.3219, -33.8635) -> (-11.3219, -36.8807)
  line L559 (-13.9349, -32.3549) -> (-11.3219, -33.8635)
  line L560 (-16.5478, -28.8807) -> (-16.5478, -25.8635)
  line L561 (-13.9349, -30.3893) -> (-16.5478, -28.8807)
  line L562 (-16.5478, -33.8635) -> (-13.9349, -32.3549)
  line L563 (-16.5478, -36.8807) -> (-16.5478, -33.8635)
  line L564 (-20.8631, -26.3893) -> (-23.476, -24.8807) construction
  line L565 (-18.2501, -21.8635) -> (-18.2501, -24.8807)
  line L566 (-18.2501, -29.8635) -> (-18.2501, -32.8807) construction
  line L567 (-18.2501, -32.8807) -> (-20.8631, -34.3893) construction
  line L568 (-20.8631, -20.3549) -> (-18.2501, -21.8635) construction
  line L569 (-20.8631, -28.3549) -> (-18.2501, -29.8635) construction
  line L570 (-23.476, -29.8635) -> (-20.8631, -28.3549) construction
  line L571 (-23.476, -24.8807) -> (-23.476, -21.8635)
  line L572 (-23.476, -21.8635) -> (-20.8631, -20.3549) construction
  line L573 (-18.2501, -37.8635) -> (-18.2501, -40.8807) construction
  line L574 (-20.8631, -36.3549) -> (-18.2501, -37.8635) construction
  line L575 (-18.2501, -40.8807) -> (-20.8631, -42.3893) construction
  line L576 (-23.476, -32.8807) -> (-23.476, -29.8635)
  line L577 (-20.8631, -34.3893) -> (-23.476, -32.8807) construction
  line L578 (-23.476, -37.8635) -> (-20.8631, -36.3549) construction
  line L579 (-23.476, -40.8807) -> (-23.476, -37.8635)
  line L580 (-20.8631, -42.3893) -> (-23.476, -40.8807) construction
  line L581 (-11.3219, -36.8807) -> (-13.9349, -38.3893)
  line L582 (-13.9349, -38.3893) -> (-16.5478, -36.8807)
  line L583 (-11.3219, -44.8807) -> (-13.9349, -46.3893)
  line L584 (-11.3219, -41.8635) -> (-11.3219, -44.8807)
  line L585 (-13.9349, -40.3549) -> (-11.3219, -41.8635)
  line L586 (-16.5478, -41.8635) -> (-13.9349, -40.3549)
  line L587 (-16.5478, -44.8807) -> (-16.5478, -41.8635)
  line L588 (-13.9349, -46.3893) -> (-16.5478, -44.8807)
  line L589 (-20.8631, -44.3549) -> (-18.2501, -45.8635) construction
  line L590 (-11.3219, -4.8807) -> (-13.9349, -6.3893)
  line L591 (-13.9349, -6.3893) -> (-16.5478, -4.8807)
  line L592 (-11.3219, -1.8635) -> (-11.3219, -4.8807)
  line L593 (-16.5478, -4.8807) -> (-16.5478, -1.8635)
  line L594 (-13.9349, -0.3549) -> (-11.3219, -1.8635) construction
  line L595 (-16.5478, -1.8635) -> (-13.9349, -0.3549) construction
  line L596 (-9.476, -16.8807) -> (-9.476, -13.8635)
  line L597 (-9.476, -8.8807) -> (-9.476, -5.8635)
  line L598 (-23.476, -45.8635) -> (-20.8631, -44.3549) construction
  line L599 (-23.476, -48.8807) -> (-23.476, -45.8635)
  line L600 (-18.2501, -45.8635) -> (-18.2501, -48.8807) construction
  line L601 (-18.2501, -48.8807) -> (-20.8631, -50.3893) construction
  line L602 (-20.8631, -50.3893) -> (-23.476, -48.8807) construction
  line L603 (-23.5, -52.5) -> (-24, -52.5)
  line L604 (-24, -52.5) -> (-24, 3.5)
  line L605 (-24, 3.5) -> (-23.5, 3.5)
  point P0 (0, 3.5)
  point P1 (0, -52.5)
  point P2 (7.1369, -7.3721)
  point P3 (5.1535, -45.5)
  point P4 (9.1204, -45.5)
  point P5 (19.1535, -45.5)
  point P6 (23.1204, -45.5)
  point P7 (26.5249, -45.5)
  point P8 (29.6054, -45.5)
  point P9 (33.1535, -45.5)
  point P10 (37.1204, -45.5)
  point P11 (47.1535, -45.5)
  point P12 (51.1204, -45.5)
  point P13 (54.5, -45.4856)
  point P14 (54.5, -41.2585)
  point P15 (54.5, -37.4856)
  point P16 (54.5, -33.2585)
  point P17 (54.5, -29.4856)
  point P18 (54.5, -25.2585)
  point P19 (54.5, -21.4856)
  point P20 (54.5, -17.2585)
  point P21 (54.5, -13.4856)
  point P22 (54.5, -9.2585)
  point P23 (54.5, -5.4856)
  point P24 (53.4522, -3.5)
  point P25 (44.6781, -3.5)
  point P26 (39.4522, -3.5)
  point P27 (30.6781, -3.5)
  point P28 (25.4522, -3.5)
  point P29 (16.6781, -3.5)
  point P30 (11.4522, -3.5)
  point P31 (-10.5, -45.5)
  point P32 (-6.8631, -7.3721)
  point P33 (-24.5, -45.5)
  point P34 (-20.8631, -7.3721)
  point P35 (12.5249, -45.5)
  point P36 (15.6054, -45.5)
  point P37 (-23.5, 0.325)
  point P38 (40.5249, -45.5)
  point P39 (43.6054, -45.5)
  point P40 (-2.5478, -3.5)
  point P41 (2.6781, -3.5)
  point P42 (-16.5, -4.9083)
  point P43 (-11.3219, -3.5)
  point P44 (-16.5, -12.9083)
  point P45 (-16.5, -9.8359)
  point P46 (-12.3946, -45.5)
  point P47 (-15.4751, -45.5)
  point P48 (-4.8796, -45.5)
  point P49 (-8.8465, -45.5)
  point P50 (-1.4751, -45.5)
  point P51 (1.6054, -45.5)
  point P52 (-16.5, -44.9083)
  dimension "d16" = 7
  dimension "d17" = 7
  dimension "d18" = 51
  dimension "d21" = 8
  dimension "d24" = 8
  dimension "d29" = 8
  dimension "d36" = 8
  dimension "d43" = 14
  dimension "d48" = 10
  dimension "d50" = 7
  dimension "d53" = 14
  dimension "d60" = 0.5
  constraints: 1204 end point, 7 point on line, 6 collinear, 6 vertical, 5 horizontal, 4 point on circle, 3 perpendicular, 2 centre point, 2 tangent, 1 coincident, 1 parallel, 1169 other
  measures "d16" distance between parallel lines of L4 L8
  measures "d17" distance between parallel lines of L1 L10
  measures "d18" distance of L8.end L9.end
  measures "d21" distance of L15.end L19.start
  measures "d24" distance of L15.end L43.start
  measures "d29" distance of L43.end L73.end
  measures "d36" distance of L37.start L79.start
  measures "d43" distance of L14.end L85.start
  measures "d48" distance between parallel lines of L4 L445
  measures "d50" distance between parallel lines of L3 L448
  measures "d53" distance of L44.start L455.start
  measures "d60" distance of L447.start L603.end
extrude "Extrusion3" add sketch "Sketch2" along normal blind 3 contours L447 L454 L3 L452 L453 L2 A9 L1 A8 L0 | L603 L604 L605 L452 L3 L454 | L7 L295 L296 L221 L222 L176 L175 L219 L220 L223 L224 L149 L150 L104 L103 L147 L148 L151 L152 L67 L68 L69 L70 L71 L72 L81 L82 L451 L509 L510 L511 L512 L513 L514 L515 L524 L583 L584 L585 L586 L448 L582 L581 L558 L559 L562 L561 L556 L554 L555 L557 L538 L534 L533 L532 L540 L537 L530 L529 L531 L535 L591 L590 L592 L449 L519 L517 L516 L518 L9 L75 L78 L73 L74 L146 L141 L142 L143 L218 L213 L214 L215 L290 L285 L10 L283 L284 L241 L240 L239 L244 L249 L260 L253 L255 L257 L259 L247 L291 L292
sketch "Sketch4" plane through (-43, -28, 4) normal (-1, 0, 0) x (0, 0, 1)
  line L0 (-11.052, 2.6258) -> (-11.052, 15.282) construction
  line L1 (-11.052, 15.282) -> (-5.8454, 15.282) construction
  line L2 (-5.8454, 15.282) -> (-5.8454, 2.6258) construction
  line L3 (-5.8454, 2.6258) -> (-11.052, 2.6258) construction
  line L4 (-13.6434, 15.282) -> (-13.6434, 2.6258) construction
  line L5 (-13.6434, 2.6258) -> (-18.85, 2.6258) construction
  line L6 (-18.85, 2.6258) -> (-18.85, 15.282) construction
  line L7 (-18.85, 15.282) -> (-13.6434, 15.282) construction
  line L8 (-4.461, 16.3693) -> (-20.2344, 16.3693) construction
  line L9 (-20.2344, 1.5385) -> (-20.2344, 16.3693) construction
  line L10 (-4.461, 1.5385) -> (-20.2344, 1.5385) construction
  line L11 (-4.461, 16.3693) -> (-4.461, 1.5385) construction
  line L12 (-13.6434, 32.8209) -> (-13.6434, 21.0196) construction
  line L13 (-13.6434, 21.0196) -> (-18.85, 21.0196) construction
  line L14 (-18.85, 21.0196) -> (-18.85, 32.8209) construction
  line L15 (-18.85, 32.8209) -> (-13.6434, 32.8209) construction
  line L16 (-11.052, 21.0196) -> (-11.052, 32.8209) construction
  line L17 (-11.052, 32.8209) -> (-5.8454, 32.8209) construction
  line L18 (-5.8454, 32.8209) -> (-5.8454, 21.0196) construction
  line L19 (-5.8454, 21.0196) -> (-11.052, 21.0196) construction
  line L20 (-4.461, 34.2124) -> (-20.2344, 34.2124) construction
  line L21 (-20.2344, 19.628) -> (-20.2344, 34.2124) construction
  line L22 (-4.461, 19.628) -> (-20.2344, 19.628) construction
  line L23 (-4.461, 34.2124) -> (-4.461, 19.628) construction
  line L24 (-16.2889, 38.9752) -> (-16.2889, 51.7421) construction
  line L25 (-16.2889, 51.7421) -> (-5.9212, 51.7421) construction
  line L26 (-5.9212, 51.7421) -> (-5.9212, 38.9752) construction
  line L27 (-5.9212, 38.9752) -> (-16.2889, 38.9752) construction
  line L28 (-5.35, 37.8923) -> (-5.35, 53.4754) construction
  line L29 (-5.35, 53.4754) -> (-18.85, 53.4754) construction
  line L30 (-18.85, 37.8923) -> (-18.85, 53.4754) construction
  line L31 (-5.35, 37.8923) -> (-18.85, 37.8923) construction
  line L32 (-20.7344, 16.8693) -> (-3.961, 16.8693)
  line L33 (-3.961, 16.8693) -> (-3.961, 1.0385)
  line L34 (-3.961, 1.0385) -> (-20.7344, 1.0385)
  line L35 (-20.7344, 1.0385) -> (-20.7344, 16.8693)
  line L36 (-20.7344, 19.128) -> (-20.7344, 34.7124)
  line L37 (-20.7344, 34.7124) -> (-3.961, 34.7124)
  line L38 (-3.961, 34.7124) -> (-3.961, 19.128)
  line L39 (-3.961, 19.128) -> (-20.7344, 19.128)
  line L40 (-19.35, 37.3923) -> (-19.35, 53.9754)
  line L41 (-19.35, 53.9754) -> (-4.85, 53.9754)
  line L42 (-4.85, 53.9754) -> (-4.85, 37.3923)
  line L43 (-4.85, 37.3923) -> (-19.35, 37.3923)
  line L44 (0, 56) -> (0, 0) construction
  line L45 (0, 0) -> (3, 0) projected
  line L46 (3, 56) -> (3, 0) projected
  line L47 (0, 56) -> (3, 56) projected
  line L48 (-27.7344, -5.9615) -> (-27.7344, 23.8693)
  line L49 (3, 0) -> (-27.7344, 0)
  line L50 (-27.7344, 0) -> (-27.7344, 56)
  line L51 (-27.7344, 56) -> (3, 56)
  line L52 (3, 56) -> (3, 0)
  line L53 (-24.7344, 53) -> (-24.7344, 3)
  line L54 (0, 3) -> (0, 53)
  point P0 (-4, 28)
  dimension "d61" = 0.5
  dimension "d62" = 0.5
  dimension "d63" = 0.5
  dimension "d64" = 7
  dimension "d65" = 3
  constraints: 38 end point, 3 parallel, 1 horizontal, 1 perpendicular, 9 other
  measures "d61" distance between parallel lines of L8 L32
  measures "d62" distance between parallel lines of L22 L39
  measures "d63" distance between parallel lines of L31 L43
  measures "d64" distance between parallel lines of L35 L48
  measures "d65" distance between parallel lines of L50 L53
ref_plane "Work Plane1" through (-43, 0, -8.3672) normal (1, 0, 0) x (0, 1, 0)
sketch "Sketch5" plane through (-43, 0, -8.3672) normal (1, 0, 0) x (0, 1, 0)
  circle A0 centre (-32.1322, -3.6183) radius 1.6 projected
  circle A1 centre (32, 8.3672) radius 1.6 projected
  circle A2 centre (-32.2241, 8.1157) radius 1.6 projected
  circle A3 centre (32, -3.3672) radius 1.6 projected
  circle A4 centre (-40.5, -16.3672) radius 2.1 projected
  circle A5 centre (40.5, -16.3672) radius 2.1 projected
  circle A6 centre (40.5, 16.3672) radius 2.1 projected
  circle A7 centre (-40.5, 16.3672) radius 2.1 projected
  line L0 (-41.5, -20.3672) -> (41.5, -20.3672) projected
  arc A8 (41.5, -20.3672) -> (44.5, -17.3672) centre (41.5, -17.3672) ccw projected
  line L1 (44.5, -17.3672) -> (44.5, 17.3672) projected
  arc A9 (44.5, 17.3672) -> (41.5, 20.3672) centre (41.5, 17.3672) ccw projected
  line L2 (41.5, 20.3672) -> (-41.5, 20.3672) projected
  arc A10 (-41.5, 20.3672) -> (-44.5, 17.3672) centre (-41.5, 17.3672) ccw projected
  line L3 (-44.5, 17.3672) -> (-44.5, -17.3672) projected
  arc A11 (-44.5, -17.3672) -> (-41.5, -20.3672) centre (-41.5, -17.3672) ccw projected
  line L4 (25.9754, -6.9828) -> (25.9754, 7.5172) projected
  line L5 (9.3923, -6.9828) -> (25.9754, -6.9828) projected
  line L6 (9.3923, 7.5172) -> (9.3923, -6.9828) projected
  line L7 (25.9754, 7.5172) -> (9.3923, 7.5172) projected
  line L8 (6.7124, 8.4062) -> (-8.872, 8.4062) projected
  line L9 (6.7124, -8.3672) -> (6.7124, 8.4062) projected
  line L10 (-8.872, -8.3672) -> (6.7124, -8.3672) projected
  line L11 (-8.872, 8.4062) -> (-8.872, -8.3672) projected
  line L12 (-11.1307, -8.3672) -> (-11.1307, 8.4062) projected
  line L13 (-26.9615, -8.3672) -> (-11.1307, -8.3672) projected
  line L14 (-26.9615, 8.4062) -> (-26.9615, -8.3672) projected
  line L15 (-11.1307, 8.4062) -> (-26.9615, 8.4062) projected
  arc A12 (28.4, -3.3672) -> (35.6, -3.3672) centre (32, -3.3672) ccw
  circle A13 centre (32, 8.3672) radius 3.6 construction
  arc A14 (-35.7234, -3.3671) -> (-28.5409, -3.3671) centre (-32.1322, -3.6183) ccw
  circle A15 centre (-32.2241, 8.1157) radius 3.6 construction
  line L16 (35.6, -3.3672) -> (35.6, 8.3672)
  line L17 (28.4, -3.3672) -> (28.4, 8.3672)
  line L18 (-28.5409, -3.3671) -> (-28.6242, 8.1417)
  line L19 (-35.7234, -3.3671) -> (-35.8239, 8.0841)
  line L20 (28, 15.3672) -> (35.6, 15.3672)
  line L21 (35.6, 15.3672) -> (35.6, 8.3672)
  line L22 (-27.7519, 15.3672) -> (-35.8239, 15.3672)
  line L23 (-35.8239, 15.3672) -> (-35.8239, 8.0841)
  line L24 (-28, 12.3672) -> (-28, 15.3672) projected
  line L25 (-28, 12.3672) -> (-28.6242, 8.1417)
  line L26 (28, 12.3672) -> (28, 15.3672) projected
  line L27 (28, 12.3672) -> (28.4, 8.3672)
  point P0 (0, 8.3672)
  dimension "d66" = 2
  dimension "d67" = 2
  dimension "d68" = 2
  dimension "d69" = 2
  constraints: 20 end point, 8 point on circle, 4 centre point, 4 tangent, 2 perpendicular, 2 point on line, 1 horizontal, 1 vertical
  measures "d66" radial gap between concentric circles of A3 A12
  measures "d67" radial gap between concentric circles of A1 A13
  measures "d68" radial gap between concentric circles of A0 A14
  measures "d69" radial gap between concentric circles of A2 A15
extrude "Extrusion4" add sketch "Sketch5" along normal blind 6 contours L17 L27 L26 L20 L21 L16 A12 | L19 L23 L22 L24 L25 L18 A14